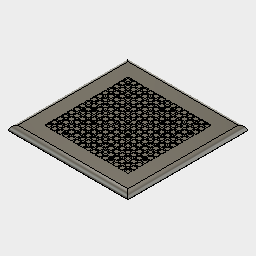
scrabble_board (Autodesk Fusion 360 design; units mm, degrees)
Autodesk Fusion 360 part; units mm, degrees
(part 1 of 6)
sketch "Sketch1" plane through (0, 0, 0) normal (0, 1, 0) x (1, 0, 0)
  line L0 (254, -254) -> (-254, -254)
  line L1 (-254, -254) -> (-254, 254)
  line L2 (-254, 254) -> (254, 254)
  line L3 (254, 254) -> (254, -254)
  line L4 (254, -254) -> (-254, 254) construction
  line L5 (-254, -254) -> (254, 254) construction
  arc A0 (-65.675, -33.5) -> (-62.5, -30.325) centre (-65.675, -30.325) ccw
  line L6 (-65.675, -33.5) -> (-78.325, -33.5)
  dimension "d1" = 508
  dimension "d2" = 508
  constraint perpendicular L0 L1
  constraint parallel L0 L2
  constraint parallel L1 L3
  constraint horizontal L0
  constraint coincident L4 origin
  constraint coincident L5 origin
extrude "Extrude1" add sketch "Sketch1" along normal blind 20.5994
sketch "Sketch2" plane through (0, 20.5994, 0) normal (0, 1, 0) x (-1, 0, 0)
  line L0 (-254, -254) -> (254, -254)
  line L1 (254, -254) -> (254, 254)
  line L2 (254, 254) -> (-254, 254)
  line L3 (-254, 254) -> (-254, -254)
  line L4 (-6.325, 9.5) -> (6.325, 9.5)
  line L5 (9.5, 6.325) -> (9.5, -6.325)
  line L6 (6.325, -9.5) -> (-6.325, -9.5)
  line L7 (-9.5, -6.325) -> (-9.5, 6.325)
  line L8 (-9.5, 9.5) -> (9.5, -9.5) construction
  line L9 (9.5, 9.5) -> (-9.5, -9.5) construction
  arc A0 (6.325, -9.5) -> (9.5, -6.325) centre (6.325, -6.325) ccw
  arc A1 (-9.5, -6.325) -> (-6.325, -9.5) centre (-6.325, -6.325) ccw
  arc A2 (-6.325, 9.5) -> (-9.5, 6.325) centre (-6.325, 6.325) ccw
  arc A3 (9.5, 6.325) -> (6.325, 9.5) centre (6.325, 6.325) ccw
  arc A4 (-161.675, -177.5) -> (-158.5, -174.325) centre (-161.675, -174.325) ccw
  line L10 (-177.5, -174.325) -> (-177.5, -161.675)
  line L11 (-158.5, -161.675) -> (-158.5, -174.325)
  line L12 (-158.5, -158.5) -> (-177.5, -177.5) construction
  arc A5 (-174.325, -158.5) -> (-177.5, -161.675) centre (-174.325, -161.675) ccw
  arc A6 (-158.5, -161.675) -> (-161.675, -158.5) centre (-161.675, -161.675) ccw
  line L13 (-161.675, -177.5) -> (-174.325, -177.5)
  line L14 (-174.325, -158.5) -> (-161.675, -158.5)
  arc A7 (-177.5, -174.325) -> (-174.325, -177.5) centre (-174.325, -174.325) ccw
  line L15 (-177.5, -158.5) -> (-158.5, -177.5) construction
  arc A8 (-137.675, -177.5) -> (-134.5, -174.325) centre (-137.675, -174.325) ccw
  line L16 (-153.5, -174.325) -> (-153.5, -161.675)
  line L17 (-134.5, -161.675) -> (-134.5, -174.325)
  line L18 (-134.5, -158.5) -> (-153.5, -177.5) construction
  arc A9 (-150.325, -158.5) -> (-153.5, -161.675) centre (-150.325, -161.675) ccw
  arc A10 (-134.5, -161.675) -> (-137.675, -158.5) centre (-137.675, -161.675) ccw
  line L19 (-137.675, -177.5) -> (-150.325, -177.5)
  line L20 (-150.325, -158.5) -> (-137.675, -158.5)
  arc A11 (-153.5, -174.325) -> (-150.325, -177.5) centre (-150.325, -174.325) ccw
  line L21 (-153.5, -158.5) -> (-134.5, -177.5) construction
  arc A12 (-113.675, -177.5) -> (-110.5, -174.325) centre (-113.675, -174.325) ccw
  line L22 (-129.5, -174.325) -> (-129.5, -161.675)
  line L23 (-110.5, -161.675) -> (-110.5, -174.325)
  line L24 (-110.5, -158.5) -> (-129.5, -177.5) construction
  arc A13 (-126.325, -158.5) -> (-129.5, -161.675) centre (-126.325, -161.675) ccw
  arc A14 (-110.5, -161.675) -> (-113.675, -158.5) centre (-113.675, -161.675) ccw
  line L25 (-113.675, -177.5) -> (-126.325, -177.5)
  line L26 (-126.325, -158.5) -> (-113.675, -158.5)
  arc A15 (-129.5, -174.325) -> (-126.325, -177.5) centre (-126.325, -174.325) ccw
  line L27 (-129.5, -158.5) -> (-110.5, -177.5) construction
  arc A16 (-89.675, -177.5) -> (-86.5, -174.325) centre (-89.675, -174.325) ccw
  line L28 (-105.5, -174.325) -> (-105.5, -161.675)
  line L29 (-86.5, -161.675) -> (-86.5, -174.325)
  line L30 (-86.5, -158.5) -> (-105.5, -177.5) construction
  arc A17 (-102.325, -158.5) -> (-105.5, -161.675) centre (-102.325, -161.675) ccw
  arc A18 (-86.5, -161.675) -> (-89.675, -158.5) centre (-89.675, -161.675) ccw
  line L31 (-89.675, -177.5) -> (-102.325, -177.5)
  line L32 (-102.325, -158.5) -> (-89.675, -158.5)
  arc A19 (-105.5, -174.325) -> (-102.325, -177.5) centre (-102.325, -174.325) ccw
  line L33 (-105.5, -158.5) -> (-86.5, -177.5) construction
  arc A20 (-65.675, -177.5) -> (-62.5, -174.325) centre (-65.675, -174.325) ccw
  line L34 (-81.5, -174.325) -> (-81.5, -161.675)
  line L35 (-62.5, -161.675) -> (-62.5, -174.325)
  line L36 (-62.5, -158.5) -> (-81.5, -177.5) construction
  arc A21 (-78.325, -158.5) -> (-81.5, -161.675) centre (-78.325, -161.675) ccw
  arc A22 (-62.5, -161.675) -> (-65.675, -158.5) centre (-65.675, -161.675) ccw
  line L37 (-65.675, -177.5) -> (-78.325, -177.5)
  line L38 (-78.325, -158.5) -> (-65.675, -158.5)
  arc A23 (-81.5, -174.325) -> (-78.325, -177.5) centre (-78.325, -174.325) ccw
  line L39 (-81.5, -158.5) -> (-62.5, -177.5) construction
  arc A24 (-41.675, -177.5) -> (-38.5, -174.325) centre (-41.675, -174.325) ccw
  line L40 (-57.5, -174.325) -> (-57.5, -161.675)
  line L41 (-38.5, -161.675) -> (-38.5, -174.325)
  line L42 (-38.5, -158.5) -> (-57.5, -177.5) construction
  arc A25 (-54.325, -158.5) -> (-57.5, -161.675) centre (-54.325, -161.675) ccw
  arc A26 (-38.5, -161.675) -> (-41.675, -158.5) centre (-41.675, -161.675) ccw
  line L43 (-41.675, -177.5) -> (-54.325, -177.5)
  line L44 (-54.325, -158.5) -> (-41.675, -158.5)
  arc A27 (-57.5, -174.325) -> (-54.325, -177.5) centre (-54.325, -174.325) ccw
  line L45 (-57.5, -158.5) -> (-38.5, -177.5) construction
  arc A28 (-17.675, -177.5) -> (-14.5, -174.325) centre (-17.675, -174.325) ccw
  line L46 (-33.5, -174.325) -> (-33.5, -161.675)
  line L47 (-14.5, -161.675) -> (-14.5, -174.325)
  line L48 (-14.5, -158.5) -> (-33.5, -177.5) construction
  arc A29 (-30.325, -158.5) -> (-33.5, -161.675) centre (-30.325, -161.675) ccw
  arc A30 (-14.5, -161.675) -> (-17.675, -158.5) centre (-17.675, -161.675) ccw
  line L49 (-17.675, -177.5) -> (-30.325, -177.5)
  line L50 (-30.325, -158.5) -> (-17.675, -158.5)
  arc A31 (-33.5, -174.325) -> (-30.325, -177.5) centre (-30.325, -174.325) ccw
  line L51 (-33.5, -158.5) -> (-14.5, -177.5) construction
  arc A32 (6.325, -177.5) -> (9.5, -174.325) centre (6.325, -174.325) ccw
  line L52 (-9.5, -174.325) -> (-9.5, -161.675)
  line L53 (9.5, -161.675) -> (9.5, -174.325)
  line L54 (9.5, -158.5) -> (-9.5, -177.5) construction
  arc A33 (-6.325, -158.5) -> (-9.5, -161.675) centre (-6.325, -161.675) ccw
  arc A34 (9.5, -161.675) -> (6.325, -158.5) centre (6.325, -161.675) ccw
  line L55 (6.325, -177.5) -> (-6.325, -177.5)
  line L56 (-6.325, -158.5) -> (6.325, -158.5)
  arc A35 (-9.5, -174.325) -> (-6.325, -177.5) centre (-6.325, -174.325) ccw
  line L57 (-9.5, -158.5) -> (9.5, -177.5) construction
  arc A36 (30.325, -177.5) -> (33.5, -174.325) centre (30.325, -174.325) ccw
  line L58 (14.5, -174.325) -> (14.5, -161.675)
  line L59 (33.5, -161.675) -> (33.5, -174.325)
  line L60 (33.5, -158.5) -> (14.5, -177.5) construction
  arc A37 (17.675, -158.5) -> (14.5, -161.675) centre (17.675, -161.675) ccw
  arc A38 (33.5, -161.675) -> (30.325, -158.5) centre (30.325, -161.675) ccw
  line L61 (30.325, -177.5) -> (17.675, -177.5)
  line L62 (17.675, -158.5) -> (30.325, -158.5)
  arc A39 (14.5, -174.325) -> (17.675, -177.5) centre (17.675, -174.325) ccw
  line L63 (14.5, -158.5) -> (33.5, -177.5) construction
  arc A40 (54.325, -177.5) -> (57.5, -174.325) centre (54.325, -174.325) ccw
  line L64 (38.5, -174.325) -> (38.5, -161.675)
  line L65 (57.5, -161.675) -> (57.5, -174.325)
  line L66 (57.5, -158.5) -> (38.5, -177.5) construction
  arc A41 (41.675, -158.5) -> (38.5, -161.675) centre (41.675, -161.675) ccw
  arc A42 (57.5, -161.675) -> (54.325, -158.5) centre (54.325, -161.675) ccw
  line L67 (54.325, -177.5) -> (41.675, -177.5)
  line L68 (41.675, -158.5) -> (54.325, -158.5)
  arc A43 (38.5, -174.325) -> (41.675, -177.5) centre (41.675, -174.325) ccw
  line L69 (38.5, -158.5) -> (57.5, -177.5) construction
  arc A44 (78.325, -177.5) -> (81.5, -174.325) centre (78.325, -174.325) ccw
  line L70 (62.5, -174.325) -> (62.5, -161.675)
  line L71 (81.5, -161.675) -> (81.5, -174.325)
  line L72 (81.5, -158.5) -> (62.5, -177.5) construction
  arc A45 (65.675, -158.5) -> (62.5, -161.675) centre (65.675, -161.675) ccw
  arc A46 (81.5, -161.675) -> (78.325, -158.5) centre (78.325, -161.675) ccw
  line L73 (78.325, -177.5) -> (65.675, -177.5)
  line L74 (65.675, -158.5) -> (78.325, -158.5)
  arc A47 (62.5, -174.325) -> (65.675, -177.5) centre (65.675, -174.325) ccw
  line L75 (62.5, -158.5) -> (81.5, -177.5) construction
  arc A48 (102.325, -177.5) -> (105.5, -174.325) centre (102.325, -174.325) ccw
  line L76 (86.5, -174.325) -> (86.5, -161.675)
  line L77 (105.5, -161.675) -> (105.5, -174.325)
  line L78 (105.5, -158.5) -> (86.5, -177.5) construction
  arc A49 (89.675, -158.5) -> (86.5, -161.675) centre (89.675, -161.675) ccw
  arc A50 (105.5, -161.675) -> (102.325, -158.5) centre (102.325, -161.675) ccw
  line L79 (102.325, -177.5) -> (89.675, -177.5)
  line L80 (89.675, -158.5) -> (102.325, -158.5)
  arc A51 (86.5, -174.325) -> (89.675, -177.5) centre (89.675, -174.325) ccw
  line L81 (86.5, -158.5) -> (105.5, -177.5) construction
  arc A52 (126.325, -177.5) -> (129.5, -174.325) centre (126.325, -174.325) ccw
  line L82 (110.5, -174.325) -> (110.5, -161.675)
  line L83 (129.5, -161.675) -> (129.5, -174.325)
  line L84 (129.5, -158.5) -> (110.5, -177.5) construction
  arc A53 (113.675, -158.5) -> (110.5, -161.675) centre (113.675, -161.675) ccw
  arc A54 (129.5, -161.675) -> (126.325, -158.5) centre (126.325, -161.675) ccw
  line L85 (126.325, -177.5) -> (113.675, -177.5)
  line L86 (113.675, -158.5) -> (126.325, -158.5)
  arc A55 (110.5, -174.325) -> (113.675, -177.5) centre (113.675, -174.325) ccw
  line L87 (110.5, -158.5) -> (129.5, -177.5) construction
  arc A56 (150.325, -177.5) -> (153.5, -174.325) centre (150.325, -174.325) ccw
  line L88 (134.5, -174.325) -> (134.5, -161.675)
  line L89 (153.5, -161.675) -> (153.5, -174.325)
  line L90 (153.5, -158.5) -> (134.5, -177.5) construction
  arc A57 (137.675, -158.5) -> (134.5, -161.675) centre (137.675, -161.675) ccw
  arc A58 (153.5, -161.675) -> (150.325, -158.5) centre (150.325, -161.675) ccw
  line L91 (150.325, -177.5) -> (137.675, -177.5)
  line L92 (137.675, -158.5) -> (150.325, -158.5)
  arc A59 (134.5, -174.325) -> (137.675, -177.5) centre (137.675, -174.325) ccw
  line L93 (134.5, -158.5) -> (153.5, -177.5) construction
  arc A60 (174.325, -177.5) -> (177.5, -174.325) centre (174.325, -174.325) ccw
  line L94 (158.5, -174.325) -> (158.5, -161.675)
  line L95 (177.5, -161.675) -> (177.5, -174.325)
  line L96 (177.5, -158.5) -> (158.5, -177.5) construction
  arc A61 (161.675, -158.5) -> (158.5, -161.675) centre (161.675, -161.675) ccw
  arc A62 (177.5, -161.675) -> (174.325, -158.5) centre (174.325, -161.675) ccw
  line L97 (174.325, -177.5) -> (161.675, -177.5)
  line L98 (161.675, -158.5) -> (174.325, -158.5)
  arc A63 (158.5, -174.325) -> (161.675, -177.5) centre (161.675, -174.325) ccw
  line L99 (158.5, -158.5) -> (177.5, -177.5) construction
  arc A64 (-161.675, -153.5) -> (-158.5, -150.325) centre (-161.675, -150.325) ccw
  line L100 (-177.5, -150.325) -> (-177.5, -137.675)
  line L101 (-158.5, -137.675) -> (-158.5, -150.325)
  line L102 (-158.5, -134.5) -> (-177.5, -153.5) construction
  arc A65 (-174.325, -134.5) -> (-177.5, -137.675) centre (-174.325, -137.675) ccw
  arc A66 (-158.5, -137.675) -> (-161.675, -134.5) centre (-161.675, -137.675) ccw
  line L103 (-161.675, -153.5) -> (-174.325, -153.5)
  line L104 (-174.325, -134.5) -> (-161.675, -134.5)
  arc A67 (-177.5, -150.325) -> (-174.325, -153.5) centre (-174.325, -150.325) ccw
  line L105 (-177.5, -134.5) -> (-158.5, -153.5) construction
  arc A68 (-137.675, -153.5) -> (-134.5, -150.325) centre (-137.675, -150.325) ccw
  line L106 (-153.5, -150.325) -> (-153.5, -137.675)
  line L107 (-134.5, -137.675) -> (-134.5, -150.325)
  line L108 (-134.5, -134.5) -> (-153.5, -153.5) construction
  arc A69 (-150.325, -134.5) -> (-153.5, -137.675) centre (-150.325, -137.675) ccw
  arc A70 (-134.5, -137.675) -> (-137.675, -134.5) centre (-137.675, -137.675) ccw
  line L109 (-137.675, -153.5) -> (-150.325, -153.5)
  line L110 (-150.325, -134.5) -> (-137.675, -134.5)
  arc A71 (-153.5, -150.325) -> (-150.325, -153.5) centre (-150.325, -150.325) ccw
  line L111 (-153.5, -134.5) -> (-134.5, -153.5) construction
  arc A72 (-113.675, -153.5) -> (-110.5, -150.325) centre (-113.675, -150.325) ccw
  line L112 (-129.5, -150.325) -> (-129.5, -137.675)
  line L113 (-110.5, -137.675) -> (-110.5, -150.325)
  line L114 (-110.5, -134.5) -> (-129.5, -153.5) construction
  arc A73 (-126.325, -134.5) -> (-129.5, -137.675) centre (-126.325, -137.675) ccw
  arc A74 (-110.5, -137.675) -> (-113.675, -134.5) centre (-113.675, -137.675) ccw
  line L115 (-113.675, -153.5) -> (-126.325, -153.5)
  line L116 (-126.325, -134.5) -> (-113.675, -134.5)
  arc A75 (-129.5, -150.325) -> (-126.325, -153.5) centre (-126.325, -150.325) ccw
  line L117 (-129.5, -134.5) -> (-110.5, -153.5) construction
  arc A76 (-89.675, -153.5) -> (-86.5, -150.325) centre (-89.675, -150.325) ccw
  line L118 (-105.5, -150.325) -> (-105.5, -137.675)
  line L119 (-86.5, -137.675) -> (-86.5, -150.325)
  line L120 (-86.5, -134.5) -> (-105.5, -153.5) construction
  arc A77 (-102.325, -134.5) -> (-105.5, -137.675) centre (-102.325, -137.675) ccw
  arc A78 (-86.5, -137.675) -> (-89.675, -134.5) centre (-89.675, -137.675) ccw
  line L121 (-89.675, -153.5) -> (-102.325, -153.5)
  line L122 (-102.325, -134.5) -> (-89.675, -134.5)
  arc A79 (-105.5, -150.325) -> (-102.325, -153.5) centre (-102.325, -150.325) ccw
  line L123 (-105.5, -134.5) -> (-86.5, -153.5) construction
  arc A80 (-65.675, -153.5) -> (-62.5, -150.325) centre (-65.675, -150.325) ccw
  line L124 (-81.5, -150.325) -> (-81.5, -137.675)
  line L125 (-62.5, -137.675) -> (-62.5, -150.325)
  line L126 (-62.5, -134.5) -> (-81.5, -153.5) construction
  arc A81 (-78.325, -134.5) -> (-81.5, -137.675) centre (-78.325, -137.675) ccw
  arc A82 (-62.5, -137.675) -> (-65.675, -134.5) centre (-65.675, -137.675) ccw
  line L127 (-65.675, -153.5) -> (-78.325, -153.5)
  line L128 (-78.325, -134.5) -> (-65.675, -134.5)
  arc A83 (-81.5, -150.325) -> (-78.325, -153.5) centre (-78.325, -150.325) ccw
  line L129 (-81.5, -134.5) -> (-62.5, -153.5) construction
  arc A84 (-41.675, -153.5) -> (-38.5, -150.325) centre (-41.675, -150.325) ccw
  line L130 (-57.5, -150.325) -> (-57.5, -137.675)
  line L131 (-38.5, -137.675) -> (-38.5, -150.325)
  line L132 (-38.5, -134.5) -> (-57.5, -153.5) construction
  arc A85 (-54.325, -134.5) -> (-57.5, -137.675) centre (-54.325, -137.675) ccw
  arc A86 (-38.5, -137.675) -> (-41.675, -134.5) centre (-41.675, -137.675) ccw
  line L133 (-41.675, -153.5) -> (-54.325, -153.5)
  line L134 (-54.325, -134.5) -> (-41.675, -134.5)
  arc A87 (-57.5, -150.325) -> (-54.325, -153.5) centre (-54.325, -150.325) ccw
  line L135 (-57.5, -134.5) -> (-38.5, -153.5) construction
  arc A88 (-17.675, -153.5) -> (-14.5, -150.325) centre (-17.675, -150.325) ccw
  line L136 (-33.5, -150.325) -> (-33.5, -137.675)
  line L137 (-14.5, -137.675) -> (-14.5, -150.325)
  line L138 (-14.5, -134.5) -> (-33.5, -153.5) construction
  arc A89 (-30.325, -134.5) -> (-33.5, -137.675) centre (-30.325, -137.675) ccw
  arc A90 (-14.5, -137.675) -> (-17.675, -134.5) centre (-17.675, -137.675) ccw
  line L139 (-17.675, -153.5) -> (-30.325, -153.5)
  line L140 (-30.325, -134.5) -> (-17.675, -134.5)
  arc A91 (-33.5, -150.325) -> (-30.325, -153.5) centre (-30.325, -150.325) ccw
  line L141 (-33.5, -134.5) -> (-14.5, -153.5) construction
  arc A92 (6.325, -153.5) -> (9.5, -150.325) centre (6.325, -150.325) ccw
  line L142 (-9.5, -150.325) -> (-9.5, -137.675)
  line L143 (9.5, -137.675) -> (9.5, -150.325)
  line L144 (9.5, -134.5) -> (-9.5, -153.5) construction
  arc A93 (-6.325, -134.5) -> (-9.5, -137.675) centre (-6.325, -137.675) ccw
  arc A94 (9.5, -137.675) -> (6.325, -134.5) centre (6.325, -137.675) ccw
  line L145 (6.325, -153.5) -> (-6.325, -153.5)
  line L146 (-6.325, -134.5) -> (6.325, -134.5)
  arc A95 (-9.5, -150.325) -> (-6.325, -153.5) centre (-6.325, -150.325) ccw
  line L147 (-9.5, -134.5) -> (9.5, -153.5) construction
  arc A96 (30.325, -153.5) -> (33.5, -150.325) centre (30.325, -150.325) ccw
  line L148 (14.5, -150.325) -> (14.5, -137.675)
  line L149 (33.5, -137.675) -> (33.5, -150.325)
  line L150 (33.5, -134.5) -> (14.5, -153.5) construction
  arc A97 (17.675, -134.5) -> (14.5, -137.675) centre (17.675, -137.675) ccw
  arc A98 (33.5, -137.675) -> (30.325, -134.5) centre (30.325, -137.675) ccw
  line L151 (30.325, -153.5) -> (17.675, -153.5)
  line L152 (17.675, -134.5) -> (30.325, -134.5)
  arc A99 (14.5, -150.325) -> (17.675, -153.5) centre (17.675, -150.325) ccw
  line L153 (14.5, -134.5) -> (33.5, -153.5) construction
  arc A100 (54.325, -153.5) -> (57.5, -150.325) centre (54.325, -150.325) ccw
  line L154 (38.5, -150.325) -> (38.5, -137.675)
  line L155 (57.5, -137.675) -> (57.5, -150.325)
  line L156 (57.5, -134.5) -> (38.5, -153.5) construction
  arc A101 (41.675, -134.5) -> (38.5, -137.675) centre (41.675, -137.675) ccw
  arc A102 (57.5, -137.675) -> (54.325, -134.5) centre (54.325, -137.675) ccw
  line L157 (54.325, -153.5) -> (41.675, -153.5)
  line L158 (41.675, -134.5) -> (54.325, -134.5)
  arc A103 (38.5, -150.325) -> (41.675, -153.5) centre (41.675, -150.325) ccw
  line L159 (38.5, -134.5) -> (57.5, -153.5) construction
  arc A104 (78.325, -153.5) -> (81.5, -150.325) centre (78.325, -150.325) ccw
  line L160 (62.5, -150.325) -> (62.5, -137.675)
  line L161 (81.5, -137.675) -> (81.5, -150.325)
  line L162 (81.5, -134.5) -> (62.5, -153.5) construction
  arc A105 (65.675, -134.5) -> (62.5, -137.675) centre (65.675, -137.675) ccw
  arc A106 (81.5, -137.675) -> (78.325, -134.5) centre (78.325, -137.675) ccw
  line L163 (78.325, -153.5) -> (65.675, -153.5)
  line L164 (65.675, -134.5) -> (78.325, -134.5)
  arc A107 (62.5, -150.325) -> (65.675, -153.5) centre (65.675, -150.325) ccw
  line L165 (62.5, -134.5) -> (81.5, -153.5) construction
  arc A108 (102.325, -153.5) -> (105.5, -150.325) centre (102.325, -150.325) ccw
  line L166 (86.5, -150.325) -> (86.5, -137.675)
  line L167 (105.5, -137.675) -> (105.5, -150.325)
  line L168 (105.5, -134.5) -> (86.5, -153.5) construction
  arc A109 (89.675, -134.5) -> (86.5, -137.675) centre (89.675, -137.675) ccw
  arc A110 (105.5, -137.675) -> (102.325, -134.5) centre (102.325, -137.675) ccw
  line L169 (102.325, -153.5) -> (89.675, -153.5)
  line L170 (89.675, -134.5) -> (102.325, -134.5)
  arc A111 (86.5, -150.325) -> (89.675, -153.5) centre (89.675, -150.325) ccw
  line L171 (86.5, -134.5) -> (105.5, -153.5) construction
  arc A112 (126.325, -153.5) -> (129.5, -150.325) centre (126.325, -150.325) ccw
  line L172 (110.5, -150.325) -> (110.5, -137.675)
  line L173 (129.5, -137.675) -> (129.5, -150.325)
  line L174 (129.5, -134.5) -> (110.5, -153.5) construction
  arc A113 (113.675, -134.5) -> (110.5, -137.675) centre (113.675, -137.675) ccw
  arc A114 (129.5, -137.675) -> (126.325, -134.5) centre (126.325, -137.675) ccw
  line L175 (126.325, -153.5) -> (113.675, -153.5)
  line L176 (113.675, -134.5) -> (126.325, -134.5)
  arc A115 (110.5, -150.325) -> (113.675, -153.5) centre (113.675, -150.325) ccw
  line L177 (110.5, -134.5) -> (129.5, -153.5) construction
  arc A116 (150.325, -153.5) -> (153.5, -150.325) centre (150.325, -150.325) ccw
  line L178 (134.5, -150.325) -> (134.5, -137.675)
  line L179 (153.5, -137.675) -> (153.5, -150.325)
  line L180 (153.5, -134.5) -> (134.5, -153.5) construction
  arc A117 (137.675, -134.5) -> (134.5, -137.675) centre (137.675, -137.675) ccw
  arc A118 (153.5, -137.675) -> (150.325, -134.5) centre (150.325, -137.675) ccw
  line L181 (150.325, -153.5) -> (137.675, -153.5)
  line L182 (137.675, -134.5) -> (150.325, -134.5)
  arc A119 (134.5, -150.325) -> (137.675, -153.5) centre (137.675, -150.325) ccw
  line L183 (134.5, -134.5) -> (153.5, -153.5) construction
  arc A120 (174.325, -153.5) -> (177.5, -150.325) centre (174.325, -150.325) ccw
  line L184 (158.5, -150.325) -> (158.5, -137.675)
  line L185 (177.5, -137.675) -> (177.5, -150.325)
  line L186 (177.5, -134.5) -> (158.5, -153.5) construction
  arc A121 (161.675, -134.5) -> (158.5, -137.675) centre (161.675, -137.675) ccw
  arc A122 (177.5, -137.675) -> (174.325, -134.5) centre (174.325, -137.675) ccw
  line L187 (174.325, -153.5) -> (161.675, -153.5)
  line L188 (161.675, -134.5) -> (174.325, -134.5)
  arc A123 (158.5, -150.325) -> (161.675, -153.5) centre (161.675, -150.325) ccw
  line L189 (158.5, -134.5) -> (177.5, -153.5) construction
  arc A124 (-161.675, -129.5) -> (-158.5, -126.325) centre (-161.675, -126.325) ccw
  line L190 (-177.5, -126.325) -> (-177.5, -113.675)
  line L191 (-158.5, -113.675) -> (-158.5, -126.325)
  line L192 (-158.5, -110.5) -> (-177.5, -129.5) construction
  arc A125 (-174.325, -110.5) -> (-177.5, -113.675) centre (-174.325, -113.675) ccw
  arc A126 (-158.5, -113.675) -> (-161.675, -110.5) centre (-161.675, -113.675) ccw
  line L193 (-161.675, -129.5) -> (-174.325, -129.5)
  line L194 (-174.325, -110.5) -> (-161.675, -110.5)
  arc A127 (-177.5, -126.325) -> (-174.325, -129.5) centre (-174.325, -126.325) ccw
  line L195 (-177.5, -110.5) -> (-158.5, -129.5) construction
  arc A128 (-137.675, -129.5) -> (-134.5, -126.325) centre (-137.675, -126.325) ccw
  line L196 (-153.5, -126.325) -> (-153.5, -113.675)
  line L197 (-134.5, -113.675) -> (-134.5, -126.325)
  line L198 (-134.5, -110.5) -> (-153.5, -129.5) construction
  arc A129 (-150.325, -110.5) -> (-153.5, -113.675) centre (-150.325, -113.675) ccw
  arc A130 (-134.5, -113.675) -> (-137.675, -110.5) centre (-137.675, -113.675) ccw
  line L199 (-137.675, -129.5) -> (-150.325, -129.5)
  line L200 (-150.325, -110.5) -> (-137.675, -110.5)
  arc A131 (-153.5, -126.325) -> (-150.325, -129.5) centre (-150.325, -126.325) ccw
  line L201 (-153.5, -110.5) -> (-134.5, -129.5) construction
  arc A132 (-113.675, -129.5) -> (-110.5, -126.325) centre (-113.675, -126.325) ccw
  line L202 (-129.5, -126.325) -> (-129.5, -113.675)
  line L203 (-110.5, -113.675) -> (-110.5, -126.325)
  line L204 (-110.5, -110.5) -> (-129.5, -129.5) construction
  arc A133 (-126.325, -110.5) -> (-129.5, -113.675) centre (-126.325, -113.675) ccw
  arc A134 (-110.5, -113.675) -> (-113.675, -110.5) centre (-113.675, -113.675) ccw
  line L205 (-113.675, -129.5) -> (-126.325, -129.5)
  line L206 (-126.325, -110.5) -> (-113.675, -110.5)
  arc A135 (-129.5, -126.325) -> (-126.325, -129.5) centre (-126.325, -126.325) ccw
  line L207 (-129.5, -110.5) -> (-110.5, -129.5) construction
  arc A136 (-89.675, -129.5) -> (-86.5, -126.325) centre (-89.675, -126.325) ccw
  line L208 (-105.5, -126.325) -> (-105.5, -113.675)
  line L209 (-86.5, -113.675) -> (-86.5, -126.325)
  line L210 (-86.5, -110.5) -> (-105.5, -129.5) construction
  arc A137 (-102.325, -110.5) -> (-105.5, -113.675) centre (-102.325, -113.675) ccw
  arc A138 (-86.5, -113.675) -> (-89.675, -110.5) centre (-89.675, -113.675) ccw
  line L211 (-89.675, -129.5) -> (-102.325, -129.5)
  line L212 (-102.325, -110.5) -> (-89.675, -110.5)
  arc A139 (-105.5, -126.325) -> (-102.325, -129.5) centre (-102.325, -126.325) ccw
  line L213 (-105.5, -110.5) -> (-86.5, -129.5) construction
  arc A140 (-65.675, -129.5) -> (-62.5, -126.325) centre (-65.675, -126.325) ccw
  line L214 (-81.5, -126.325) -> (-81.5, -113.675)
  line L215 (-62.5, -113.675) -> (-62.5, -126.325)
  line L216 (-62.5, -110.5) -> (-81.5, -129.5) construction
  arc A141 (-78.325, -110.5) -> (-81.5, -113.675) centre (-78.325, -113.675) ccw
  arc A142 (-62.5, -113.675) -> (-65.675, -110.5) centre (-65.675, -113.675) ccw
  line L217 (-65.675, -129.5) -> (-78.325, -129.5)
  line L218 (-78.325, -110.5) -> (-65.675, -110.5)
  arc A143 (-81.5, -126.325) -> (-78.325, -129.5) centre (-78.325, -126.325) ccw
  line L219 (-81.5, -110.5) -> (-62.5, -129.5) construction
  arc A144 (-41.675, -129.5) -> (-38.5, -126.325) centre (-41.675, -126.325) ccw
  line L220 (-57.5, -126.325) -> (-57.5, -113.675)
  line L221 (-38.5, -113.675) -> (-38.5, -126.325)
  line L222 (-38.5, -110.5) -> (-57.5, -129.5) construction
  arc A145 (-54.325, -110.5) -> (-57.5, -113.675) centre (-54.325, -113.675) ccw
  arc A146 (-38.5, -113.675) -> (-41.675, -110.5) centre (-41.675, -113.675) ccw
  line L223 (-41.675, -129.5) -> (-54.325, -129.5)
  line L224 (-54.325, -110.5) -> (-41.675, -110.5)
  arc A147 (-57.5, -126.325) -> (-54.325, -129.5) centre (-54.325, -126.325) ccw
  line L225 (-57.5, -110.5) -> (-38.5, -129.5) construction
  arc A148 (-17.675, -129.5) -> (-14.5, -126.325) centre (-17.675, -126.325) ccw
  line L226 (-33.5, -126.325) -> (-33.5, -113.675)
  line L227 (-14.5, -113.675) -> (-14.5, -126.325)
  line L228 (-14.5, -110.5) -> (-33.5, -129.5) construction
  arc A149 (-30.325, -110.5) -> (-33.5, -113.675) centre (-30.325, -113.675) ccw
  arc A150 (-14.5, -113.675) -> (-17.675, -110.5) centre (-17.675, -113.675) ccw
  line L229 (-17.675, -129.5) -> (-30.325, -129.5)
  line L230 (-30.325, -110.5) -> (-17.675, -110.5)
  arc A151 (-33.5, -126.325) -> (-30.325, -129.5) centre (-30.325, -126.325) ccw
  line L231 (-33.5, -110.5) -> (-14.5, -129.5) construction
  arc A152 (6.325, -129.5) -> (9.5, -126.325) centre (6.325, -126.325) ccw
  line L232 (-9.5, -126.325) -> (-9.5, -113.675)
  line L233 (9.5, -113.675) -> (9.5, -126.325)
  line L234 (9.5, -110.5) -> (-9.5, -129.5) construction
  arc A153 (-6.325, -110.5) -> (-9.5, -113.675) centre (-6.325, -113.675) ccw
  arc A154 (9.5, -113.675) -> (6.325, -110.5) centre (6.325, -113.675) ccw
  line L235 (6.325, -129.5) -> (-6.325, -129.5)
  line L236 (-6.325, -110.5) -> (6.325, -110.5)
  arc A155 (-9.5, -126.325) -> (-6.325, -129.5) centre (-6.325, -126.325) ccw
  line L237 (-9.5, -110.5) -> (9.5, -129.5) construction
  arc A156 (30.325, -129.5) -> (33.5, -126.325) centre (30.325, -126.325) ccw
  line L238 (14.5, -126.325) -> (14.5, -113.675)
  line L239 (33.5, -113.675) -> (33.5, -126.325)
  line L240 (33.5, -110.5) -> (14.5, -129.5) construction
  arc A157 (17.675, -110.5) -> (14.5, -113.675) centre (17.675, -113.675) ccw
  arc A158 (33.5, -113.675) -> (30.325, -110.5) centre (30.325, -113.675) ccw
  line L241 (30.325, -129.5) -> (17.675, -129.5)
  line L242 (17.675, -110.5) -> (30.325, -110.5)
  arc A159 (14.5, -126.325) -> (17.675, -129.5) centre (17.675, -126.325) ccw
  line L243 (14.5, -110.5) -> (33.5, -129.5) construction
  arc A160 (54.325, -129.5) -> (57.5, -126.325) centre (54.325, -126.325) ccw
  line L244 (38.5, -126.325) -> (38.5, -113.675)
  line L245 (57.5, -113.675) -> (57.5, -126.325)
  line L246 (57.5, -110.5) -> (38.5, -129.5) construction
  arc A161 (41.675, -110.5) -> (38.5, -113.675) centre (41.675, -113.675) ccw
  arc A162 (57.5, -113.675) -> (54.325, -110.5) centre (54.325, -113.675) ccw
  line L247 (54.325, -129.5) -> (41.675, -129.5)
  line L248 (41.675, -110.5) -> (54.325, -110.5)
  arc A163 (38.5, -126.325) -> (41.675, -129.5) centre (41.675, -126.325) ccw
  line L249 (38.5, -110.5) -> (57.5, -129.5) construction
  arc A164 (78.325, -129.5) -> (81.5, -126.325) centre (78.325, -126.325) ccw
  line L250 (62.5, -126.325) -> (62.5, -113.675)
  line L251 (81.5, -113.675) -> (81.5, -126.325)
  line L252 (81.5, -110.5) -> (62.5, -129.5) construction
  arc A165 (65.675, -110.5) -> (62.5, -113.675) centre (65.675, -113.675) ccw
  arc A166 (81.5, -113.675) -> (78.325, -110.5) centre (78.325, -113.675) ccw
  line L253 (78.325, -129.5) -> (65.675, -129.5)
  line L254 (65.675, -110.5) -> (78.325, -110.5)
  arc A167 (62.5, -126.325) -> (65.675, -129.5) centre (65.675, -126.325) ccw
  line L255 (62.5, -110.5) -> (81.5, -129.5) construction
  arc A168 (102.325, -129.5) -> (105.5, -126.325) centre (102.325, -126.325) ccw
  line L256 (86.5, -126.325) -> (86.5, -113.675)
  line L257 (105.5, -113.675) -> (105.5, -126.325)
  line L258 (105.5, -110.5) -> (86.5, -129.5) construction
  arc A169 (89.675, -110.5) -> (86.5, -113.675) centre (89.675, -113.675) ccw
  arc A170 (105.5, -113.675) -> (102.325, -110.5) centre (102.325, -113.675) ccw
  line L259 (102.325, -129.5) -> (89.675, -129.5)
  line L260 (89.675, -110.5) -> (102.325, -110.5)
  arc A171 (86.5, -126.325) -> (89.675, -129.5) centre (89.675, -126.325) ccw
  line L261 (86.5, -110.5) -> (105.5, -129.5) construction
  arc A172 (126.325, -129.5) -> (129.5, -126.325) centre (126.325, -126.325) ccw
  line L262 (110.5, -126.325) -> (110.5, -113.675)
  line L263 (129.5, -113.675) -> (129.5, -126.325)
  line L264 (129.5, -110.5) -> (110.5, -129.5) construction
  arc A173 (113.675, -110.5) -> (110.5, -113.675) centre (113.675, -113.675) ccw
  arc A174 (129.5, -113.675) -> (126.325, -110.5) centre (126.325, -113.675) ccw
  line L265 (126.325, -129.5) -> (113.675, -129.5)
  line L266 (113.675, -110.5) -> (126.325, -110.5)
  arc A175 (110.5, -126.325) -> (113.675, -129.5) centre (113.675, -126.325) ccw
  line L267 (110.5, -110.5) -> (129.5, -129.5) construction
  arc A176 (150.325, -129.5) -> (153.5, -126.325) centre (150.325, -126.325) ccw
  line L268 (134.5, -126.325) -> (134.5, -113.675)
  line L269 (153.5, -113.675) -> (153.5, -126.325)
  line L270 (153.5, -110.5) -> (134.5, -129.5) construction
  arc A177 (137.675, -110.5) -> (134.5, -113.675) centre (137.675, -113.675) ccw
  arc A178 (153.5, -113.675) -> (150.325, -110.5) centre (150.325, -113.675) ccw
  line L271 (150.325, -129.5) -> (137.675, -129.5)
  line L272 (137.675, -110.5) -> (150.325, -110.5)
  arc A179 (134.5, -126.325) -> (137.675, -129.5) centre (137.675, -126.325) ccw
  line L273 (134.5, -110.5) -> (153.5, -129.5) construction
  arc A180 (174.325, -129.5) -> (177.5, -126.325) centre (174.325, -126.325) ccw
  line L274 (158.5, -126.325) -> (158.5, -113.675)
  line L275 (177.5, -113.675) -> (177.5, -126.325)
  line L276 (177.5, -110.5) -> (158.5, -129.5) construction
  arc A181 (161.675, -110.5) -> (158.5, -113.675) centre (161.675, -113.675) ccw
  arc A182 (177.5, -113.675) -> (174.325, -110.5) centre (174.325, -113.675) ccw
  line L277 (174.325, -129.5) -> (161.675, -129.5)
  line L278 (161.675, -110.5) -> (174.325, -110.5)
  arc A183 (158.5, -126.325) -> (161.675, -129.5) centre (161.675, -126.325) ccw
  line L279 (158.5, -110.5) -> (177.5, -129.5) construction
  arc A184 (-161.675, -105.5) -> (-158.5, -102.325) centre (-161.675, -102.325) ccw
  line L280 (-177.5, -102.325) -> (-177.5, -89.675)
  line L281 (-158.5, -89.675) -> (-158.5, -102.325)
  line L282 (-158.5, -86.5) -> (-177.5, -105.5) construction
  arc A185 (-174.325, -86.5) -> (-177.5, -89.675) centre (-174.325, -89.675) ccw
  arc A186 (-158.5, -89.675) -> (-161.675, -86.5) centre (-161.675, -89.675) ccw
  line L283 (-161.675, -105.5) -> (-174.325, -105.5)
  line L284 (-174.325, -86.5) -> (-161.675, -86.5)
  arc A187 (-177.5, -102.325) -> (-174.325, -105.5) centre (-174.325, -102.325) ccw
  line L285 (-177.5, -86.5) -> (-158.5, -105.5) construction
  arc A188 (-137.675, -105.5) -> (-134.5, -102.325) centre (-137.675, -102.325) ccw
  line L286 (-153.5, -102.325) -> (-153.5, -89.675)
  line L287 (-134.5, -89.675) -> (-134.5, -102.325)
  line L288 (-134.5, -86.5) -> (-153.5, -105.5) construction
  arc A189 (-150.325, -86.5) -> (-153.5, -89.675) centre (-150.325, -89.675) ccw
  arc A190 (-134.5, -89.675) -> (-137.675, -86.5) centre (-137.675, -89.675) ccw
  line L289 (-137.675, -105.5) -> (-150.325, -105.5)
  line L290 (-150.325, -86.5) -> (-137.675, -86.5)
  arc A191 (-153.5, -102.325) -> (-150.325, -105.5) centre (-150.325, -102.325) ccw
  line L291 (-153.5, -86.5) -> (-134.5, -105.5) construction
  arc A192 (-113.675, -105.5) -> (-110.5, -102.325) centre (-113.675, -102.325) ccw
  line L292 (-129.5, -102.325) -> (-129.5, -89.675)
  line L293 (-110.5, -89.675) -> (-110.5, -102.325)
  line L294 (-110.5, -86.5) -> (-129.5, -105.5) construction
  arc A193 (-126.325, -86.5) -> (-129.5, -89.675) centre (-126.325, -89.675) ccw
  arc A194 (-110.5, -89.675) -> (-113.675, -86.5) centre (-113.675, -89.675) ccw
  line L295 (-113.675, -105.5) -> (-126.325, -105.5)
  line L296 (-126.325, -86.5) -> (-113.675, -86.5)
  arc A195 (-129.5, -102.325) -> (-126.325, -105.5) centre (-126.325, -102.325) ccw
  line L297 (-129.5, -86.5) -> (-110.5, -105.5) construction
  arc A196 (-89.675, -105.5) -> (-86.5, -102.325) centre (-89.675, -102.325) ccw
  line L298 (-105.5, -102.325) -> (-105.5, -89.675)
  line L299 (-86.5, -89.675) -> (-86.5, -102.325)
  line L300 (-86.5, -86.5) -> (-105.5, -105.5) construction
  arc A197 (-102.325, -86.5) -> (-105.5, -89.675) centre (-102.325, -89.675) ccw
  arc A198 (-86.5, -89.675) -> (-89.675, -86.5) centre (-89.675, -89.675) ccw
  line L301 (-89.675, -105.5) -> (-102.325, -105.5)
  line L302 (-102.325, -86.5) -> (-89.675, -86.5)
  arc A199 (-105.5, -102.325) -> (-102.325, -105.5) centre (-102.325, -102.325) ccw
  line L303 (-105.5, -86.5) -> (-86.5, -105.5) construction
  arc A200 (-65.675, -105.5) -> (-62.5, -102.325) centre (-65.675, -102.325) ccw
  line L304 (-81.5, -102.325) -> (-81.5, -89.675)
  line L305 (-62.5, -89.675) -> (-62.5, -102.325)
  line L306 (-62.5, -86.5) -> (-81.5, -105.5) construction
  arc A201 (-78.325, -86.5) -> (-81.5, -89.675) centre (-78.325, -89.675) ccw
  arc A202 (-62.5, -89.675) -> (-65.675, -86.5) centre (-65.675, -89.675) ccw
  line L307 (-65.675, -105.5) -> (-78.325, -105.5)
  line L308 (-78.325, -86.5) -> (-65.675, -86.5)
  arc A203 (-81.5, -102.325) -> (-78.325, -105.5) centre (-78.325, -102.325) ccw
  line L309 (-81.5, -86.5) -> (-62.5, -105.5) construction
  arc A204 (-41.675, -105.5) -> (-38.5, -102.325) centre (-41.675, -102.325) ccw
  line L310 (-57.5, -102.325) -> (-57.5, -89.675)
  line L311 (-38.5, -89.675) -> (-38.5, -102.325)
  line L312 (-38.5, -86.5) -> (-57.5, -105.5) construction
  arc A205 (-54.325, -86.5) -> (-57.5, -89.675) centre (-54.325, -89.675) ccw
  arc A206 (-38.5, -89.675) -> (-41.675, -86.5) centre (-41.675, -89.675) ccw
  line L313 (-41.675, -105.5) -> (-54.325, -105.5)
  line L314 (-54.325, -86.5) -> (-41.675, -86.5)
  arc A207 (-57.5, -102.325) -> (-54.325, -105.5) centre (-54.325, -102.325) ccw
  line L315 (-57.5, -86.5) -> (-38.5, -105.5) construction
  arc A208 (-17.675, -105.5) -> (-14.5, -102.325) centre (-17.675, -102.325) ccw
  line L316 (-33.5, -102.325) -> (-33.5, -89.675)
  line L317 (-14.5, -89.675) -> (-14.5, -102.325)
  line L318 (-14.5, -86.5) -> (-33.5, -105.5) construction
  arc A209 (-30.325, -86.5) -> (-33.5, -89.675) centre (-30.325, -89.675) ccw
  arc A210 (-14.5, -89.675) -> (-17.675, -86.5) centre (-17.675, -89.675) ccw
  line L319 (-17.675, -105.5) -> (-30.325, -105.5)
  line L320 (-30.325, -86.5) -> (-17.675, -86.5)
  arc A211 (-33.5, -102.325) -> (-30.325, -105.5) centre (-30.325, -102.325) ccw
  line L321 (-33.5, -86.5) -> (-14.5, -105.5) construction
  arc A212 (6.325, -105.5) -> (9.5, -102.325) centre (6.325, -102.325) ccw
  line L322 (-9.5, -102.325) -> (-9.5, -89.675)
  line L323 (9.5, -89.675) -> (9.5, -102.325)
  line L324 (9.5, -86.5) -> (-9.5, -105.5) construction
  arc A213 (-6.325, -86.5) -> (-9.5, -89.675) centre (-6.325, -89.675) ccw
  arc A214 (9.5, -89.675) -> (6.325, -86.5) centre (6.325, -89.675) ccw
  line L325 (6.325, -105.5) -> (-6.325, -105.5)
  line L326 (-6.325, -86.5) -> (6.325, -86.5)
  arc A215 (-9.5, -102.325) -> (-6.325, -105.5) centre (-6.325, -102.325) ccw
  line L327 (-9.5, -86.5) -> (9.5, -105.5) construction
  arc A216 (30.325, -105.5) -> (33.5, -102.325) centre (30.325, -102.325) ccw
  line L328 (14.5, -102.325) -> (14.5, -89.675)
  line L329 (33.5, -89.675) -> (33.5, -102.325)
  line L330 (33.5, -86.5) -> (14.5, -105.5) construction
  arc A217 (17.675, -86.5) -> (14.5, -89.675) centre (17.675, -89.675) ccw
  arc A218 (33.5, -89.675) -> (30.325, -86.5) centre (30.325, -89.675) ccw
  line L331 (30.325, -105.5) -> (17.675, -105.5)
  line L332 (17.675, -86.5) -> (30.325, -86.5)
  arc A219 (14.5, -102.325) -> (17.675, -105.5) centre (17.675, -102.325) ccw
  line L333 (14.5, -86.5) -> (33.5, -105.5) construction
  arc A220 (54.325, -105.5) -> (57.5, -102.325) centre (54.325, -102.325) ccw
  line L334 (38.5, -102.325) -> (38.5, -89.675)
  line L335 (57.5, -89.675) -> (57.5, -102.325)
  line L336 (57.5, -86.5) -> (38.5, -105.5) construction
  arc A221 (41.675, -86.5) -> (38.5, -89.675) centre (41.675, -89.675) ccw
  arc A222 (57.5, -89.675) -> (54.325, -86.5) centre (54.325, -89.675) ccw
  line L337 (54.325, -105.5) -> (41.675, -105.5)
  line L338 (41.675, -86.5) -> (54.325, -86.5)
  arc A223 (38.5, -102.325) -> (41.675, -105.5) centre (41.675, -102.325) ccw
  line L339 (38.5, -86.5) -> (57.5, -105.5) construction
  arc A224 (78.325, -105.5) -> (81.5, -102.325) centre (78.325, -102.325) ccw
  line L340 (62.5, -102.325) -> (62.5, -89.675)
  line L341 (81.5, -89.675) -> (81.5, -102.325)
  line L342 (81.5, -86.5) -> (62.5, -105.5) construction
  arc A225 (65.675, -86.5) -> (62.5, -89.675) centre (65.675, -89.675) ccw
  arc A226 (81.5, -89.675) -> (78.325, -86.5) centre (78.325, -89.675) ccw
  line L343 (78.325, -105.5) -> (65.675, -105.5)
  line L344 (65.675, -86.5) -> (78.325, -86.5)
  arc A227 (62.5, -102.325) -> (65.675, -105.5) centre (65.675, -102.325) ccw
  line L345 (62.5, -86.5) -> (81.5, -105.5) construction
  arc A228 (102.325, -105.5) -> (105.5, -102.325) centre (102.325, -102.325) ccw
  line L346 (86.5, -102.325) -> (86.5, -89.675)
  line L347 (105.5, -89.675) -> (105.5, -102.325)
  line L348 (105.5, -86.5) -> (86.5, -105.5) construction
  arc A229 (89.675, -86.5) -> (86.5, -89.675) centre (89.675, -89.675) ccw
  arc A230 (105.5, -89.675) -> (102.325, -86.5) centre (102.325, -89.675) ccw
  line L349 (102.325, -105.5) -> (89.675, -105.5)
  line L350 (89.675, -86.5) -> (102.325, -86.5)
  arc A231 (86.5, -102.325) -> (89.675, -105.5) centre (89.675, -102.325) ccw
  line L351 (86.5, -86.5) -> (105.5, -105.5) construction
  arc A232 (126.325, -105.5) -> (129.5, -102.325) centre (126.325, -102.325) ccw
  line L352 (110.5, -102.325) -> (110.5, -89.675)
  line L353 (129.5, -89.675) -> (129.5, -102.325)
  line L354 (129.5, -86.5) -> (110.5, -105.5) construction
  arc A233 (113.675, -86.5) -> (110.5, -89.675) centre (113.675, -89.675) ccw
  arc A234 (129.5, -89.675) -> (126.325, -86.5) centre (126.325, -89.675) ccw
  line L355 (126.325, -105.5) -> (113.675, -105.5)
  line L356 (113.675, -86.5) -> (126.325, -86.5)
  arc A235 (110.5, -102.325) -> (113.675, -105.5) centre (113.675, -102.325) ccw
  line L357 (110.5, -86.5) -> (129.5, -105.5) construction
  arc A236 (150.325, -105.5) -> (153.5, -102.325) centre (150.325, -102.325) ccw
  line L358 (134.5, -102.325) -> (134.5, -89.675)
  line L359 (153.5, -89.675) -> (153.5, -102.325)
  line L360 (153.5, -86.5) -> (134.5, -105.5) construction
  arc A237 (137.675, -86.5) -> (134.5, -89.675) centre (137.675, -89.675) ccw
  arc A238 (153.5, -89.675) -> (150.325, -86.5) centre (150.325, -89.675) ccw
  line L361 (150.325, -105.5) -> (137.675, -105.5)
  line L362 (137.675, -86.5) -> (150.325, -86.5)
  arc A239 (134.5, -102.325) -> (137.675, -105.5) centre (137.675, -102.325) ccw
  line L363 (134.5, -86.5) -> (153.5, -105.5) construction
  arc A240 (174.325, -105.5) -> (177.5, -102.325) centre (174.325, -102.325) ccw
  line L364 (158.5, -102.325) -> (158.5, -89.675)
  line L365 (177.5, -89.675) -> (177.5, -102.325)
  line L366 (177.5, -86.5) -> (158.5, -105.5) construction
  arc A241 (161.675, -86.5) -> (158.5, -89.675) centre (161.675, -89.675) ccw
  arc A242 (177.5, -89.675) -> (174.325, -86.5) centre (174.325, -89.675) ccw
  line L367 (174.325, -105.5) -> (161.675, -105.5)
  line L368 (161.675, -86.5) -> (174.325, -86.5)
  arc A243 (158.5, -102.325) -> (161.675, -105.5) centre (161.675, -102.325) ccw
  line L369 (158.5, -86.5) -> (177.5, -105.5) construction
  arc A244 (-161.675, -81.5) -> (-158.5, -78.325) centre (-161.675, -78.325) ccw
  line L370 (-177.5, -78.325) -> (-177.5, -65.675)
  line L371 (-158.5, -65.675) -> (-158.5, -78.325)
  line L372 (-158.5, -62.5) -> (-177.5, -81.5) construction
  arc A245 (-174.325, -62.5) -> (-177.5, -65.675) centre (-174.325, -65.675) ccw
  arc A246 (-158.5, -65.675) -> (-161.675, -62.5) centre (-161.675, -65.675) ccw
  line L373 (-161.675, -81.5) -> (-174.325, -81.5)
  line L374 (-174.325, -62.5) -> (-161.675, -62.5)
  arc A247 (-177.5, -78.325) -> (-174.325, -81.5) centre (-174.325, -78.325) ccw
  line L375 (-177.5, -62.5) -> (-158.5, -81.5) construction
  arc A248 (-137.675, -81.5) -> (-134.5, -78.325) centre (-137.675, -78.325) ccw
  line L376 (-153.5, -78.325) -> (-153.5, -65.675)
  line L377 (-134.5, -65.675) -> (-134.5, -78.325)
  line L378 (-134.5, -62.5) -> (-153.5, -81.5) construction
  arc A249 (-150.325, -62.5) -> (-153.5, -65.675) centre (-150.325, -65.675) ccw
  arc A250 (-134.5, -65.675) -> (-137.675, -62.5) centre (-137.675, -65.675) ccw
  line L379 (-137.675, -81.5) -> (-150.325, -81.5)
  line L380 (-150.325, -62.5) -> (-137.675, -62.5)
  arc A251 (-153.5, -78.325) -> (-150.325, -81.5) centre (-150.325, -78.325) ccw
  line L381 (-153.5, -62.5) -> (-134.5, -81.5) construction
  arc A252 (-113.675, -81.5) -> (-110.5, -78.325) centre (-113.675, -78.325) ccw
  line L382 (-129.5, -78.325) -> (-129.5, -65.675)
  line L383 (-110.5, -65.675) -> (-110.5, -78.325)
  line L384 (-110.5, -62.5) -> (-129.5, -81.5) construction
  arc A253 (-126.325, -62.5) -> (-129.5, -65.675) centre (-126.325, -65.675) ccw
  arc A254 (-110.5, -65.675) -> (-113.675, -62.5) centre (-113.675, -65.675) ccw
  line L385 (-113.675, -81.5) -> (-126.325, -81.5)
  line L386 (-126.325, -62.5) -> (-113.675, -62.5)
  arc A255 (-129.5, -78.325) -> (-126.325, -81.5) centre (-126.325, -78.325) ccw
  line L387 (-129.5, -62.5) -> (-110.5, -81.5) construction
  arc A256 (-89.675, -81.5) -> (-86.5, -78.325) centre (-89.675, -78.325) ccw
  line L388 (-105.5, -78.325) -> (-105.5, -65.675)
  line L389 (-86.5, -65.675) -> (-86.5, -78.325)
  line L390 (-86.5, -62.5) -> (-105.5, -81.5) construction
  arc A257 (-102.325, -62.5) -> (-105.5, -65.675) centre (-102.325, -65.675) ccw
  arc A258 (-86.5, -65.675) -> (-89.675, -62.5) centre (-89.675, -65.675) ccw
  line L391 (-89.675, -81.5) -> (-102.325, -81.5)
  line L392 (-102.325, -62.5) -> (-89.675, -62.5)
  arc A259 (-105.5, -78.325) -> (-102.325, -81.5) centre (-102.325, -78.325) ccw
  line L393 (-105.5, -62.5) -> (-86.5, -81.5) construction
  arc A260 (-65.675, -81.5) -> (-62.5, -78.325) centre (-65.675, -78.325) ccw
  line L394 (-81.5, -78.325) -> (-81.5, -65.675)
  line L395 (-62.5, -65.675) -> (-62.5, -78.325)
  line L396 (-62.5, -62.5) -> (-81.5, -81.5) construction
  arc A261 (-78.325, -62.5) -> (-81.5, -65.675) centre (-78.325, -65.675) ccw
  arc A262 (-62.5, -65.675) -> (-65.675, -62.5) centre (-65.675, -65.675) ccw
  line L397 (-65.675, -81.5) -> (-78.325, -81.5)
  line L398 (-78.325, -62.5) -> (-65.675, -62.5)
  arc A263 (-81.5, -78.325) -> (-78.325, -81.5) centre (-78.325, -78.325) ccw
  line L399 (-81.5, -62.5) -> (-62.5, -81.5) construction
  arc A264 (-41.675, -81.5) -> (-38.5, -78.325) centre (-41.675, -78.325) ccw
  line L400 (-57.5, -78.325) -> (-57.5, -65.675)
  line L401 (-38.5, -65.675) -> (-38.5, -78.325)
  line L402 (-38.5, -62.5) -> (-57.5, -81.5) construction
  arc A265 (-54.325, -62.5) -> (-57.5, -65.675) centre (-54.325, -65.675) ccw
  arc A266 (-38.5, -65.675) -> (-41.675, -62.5) centre (-41.675, -65.675) ccw
  line L403 (-41.675, -81.5) -> (-54.325, -81.5)
  line L404 (-54.325, -62.5) -> (-41.675, -62.5)
  arc A267 (-57.5, -78.325) -> (-54.325, -81.5) centre (-54.325, -78.325) ccw
  line L405 (-57.5, -62.5) -> (-38.5, -81.5) construction
  arc A268 (-17.675, -81.5) -> (-14.5, -78.325) centre (-17.675, -78.325) ccw
  line L406 (-33.5, -78.325) -> (-33.5, -65.675)
  line L407 (-14.5, -65.675) -> (-14.5, -78.325)
  line L408 (-14.5, -62.5) -> (-33.5, -81.5) construction
  arc A269 (-30.325, -62.5) -> (-33.5, -65.675) centre (-30.325, -65.675) ccw
  arc A270 (-14.5, -65.675) -> (-17.675, -62.5) centre (-17.675, -65.675) ccw
  line L409 (-17.675, -81.5) -> (-30.325, -81.5)
  line L410 (-30.325, -62.5) -> (-17.675, -62.5)
  arc A271 (-33.5, -78.325) -> (-30.325, -81.5) centre (-30.325, -78.325) ccw
  line L411 (-33.5, -62.5) -> (-14.5, -81.5) construction
  arc A272 (6.325, -81.5) -> (9.5, -78.325) centre (6.325, -78.325) ccw
  line L412 (-9.5, -78.325) -> (-9.5, -65.675)
  line L413 (9.5, -65.675) -> (9.5, -78.325)
  line L414 (9.5, -62.5) -> (-9.5, -81.5) construction
  arc A273 (-6.325, -62.5) -> (-9.5, -65.675) centre (-6.325, -65.675) ccw
  arc A274 (9.5, -65.675) -> (6.325, -62.5) centre (6.325, -65.675) ccw
  line L415 (6.325, -81.5) -> (-6.325, -81.5)
  line L416 (-6.325, -62.5) -> (6.325, -62.5)
  arc A275 (-9.5, -78.325) -> (-6.325, -81.5) centre (-6.325, -78.325) ccw
  line L417 (-9.5, -62.5) -> (9.5, -81.5) construction
  arc A276 (30.325, -81.5) -> (33.5, -78.325) centre (30.325, -78.325) ccw
  line L418 (14.5, -78.325) -> (14.5, -65.675)
  line L419 (33.5, -65.675) -> (33.5, -78.325)
  line L420 (33.5, -62.5) -> (14.5, -81.5) construction
  arc A277 (17.675, -62.5) -> (14.5, -65.675) centre (17.675, -65.675) ccw
  arc A278 (33.5, -65.675) -> (30.325, -62.5) centre (30.325, -65.675) ccw
  line L421 (30.325, -81.5) -> (17.675, -81.5)
  line L422 (17.675, -62.5) -> (30.325, -62.5)
  arc A279 (14.5, -78.325) -> (17.675, -81.5) centre (17.675, -78.325) ccw
  line L423 (14.5, -62.5) -> (33.5, -81.5) construction
  arc A280 (54.325, -81.5) -> (57.5, -78.325) centre (54.325, -78.325) ccw
  line L424 (38.5, -78.325) -> (38.5, -65.675)
  line L425 (57.5, -65.675) -> (57.5, -78.325)
  line L426 (57.5, -62.5) -> (38.5, -81.5) construction
  arc A281 (41.675, -62.5) -> (38.5, -65.675) centre (41.675, -65.675) ccw
  arc A282 (57.5, -65.675) -> (54.325, -62.5) centre (54.325, -65.675) ccw
  line L427 (54.325, -81.5) -> (41.675, -81.5)
  line L428 (41.675, -62.5) -> (54.325, -62.5)
  arc A283 (38.5, -78.325) -> (41.675, -81.5) centre (41.675, -78.325) ccw
  line L429 (38.5, -62.5) -> (57.5, -81.5) construction
  arc A284 (78.325, -81.5) -> (81.5, -78.325) centre (78.325, -78.325) ccw
  line L430 (62.5, -78.325) -> (62.5, -65.675)
  line L431 (81.5, -65.675) -> (81.5, -78.325)
  line L432 (81.5, -62.5) -> (62.5, -81.5) construction
  arc A285 (65.675, -62.5) -> (62.5, -65.675) centre (65.675, -65.675) ccw
  arc A286 (81.5, -65.675) -> (78.325, -62.5) centre (78.325, -65.675) ccw
  line L433 (78.325, -81.5) -> (65.675, -81.5)
  line L434 (65.675, -62.5) -> (78.325, -62.5)
  arc A287 (62.5, -78.325) -> (65.675, -81.5) centre (65.675, -78.325) ccw
  line L435 (62.5, -62.5) -> (81.5, -81.5) construction
  arc A288 (102.325, -81.5) -> (105.5, -78.325) centre (102.325, -78.325) ccw
  line L436 (86.5, -78.325) -> (86.5, -65.675)
  line L437 (105.5, -65.675) -> (105.5, -78.325)
  line L438 (105.5, -62.5) -> (86.5, -81.5) construction
  arc A289 (89.675, -62.5) -> (86.5, -65.675) centre (89.675, -65.675) ccw
  arc A290 (105.5, -65.675) -> (102.325, -62.5) centre (102.325, -65.675) ccw
  line L439 (102.325, -81.5) -> (89.675, -81.5)
  line L440 (89.675, -62.5) -> (102.325, -62.5)
  arc A291 (86.5, -78.325) -> (89.675, -81.5) centre (89.675, -78.325) ccw
  line L441 (86.5, -62.5) -> (105.5, -81.5) construction
  arc A292 (126.325, -81.5) -> (129.5, -78.325) centre (126.325, -78.325) ccw
  line L442 (110.5, -78.325) -> (110.5, -65.675)
  line L443 (129.5, -65.675) -> (129.5, -78.325)
  line L444 (129.5, -62.5) -> (110.5, -81.5) construction
  arc A293 (113.675, -62.5) -> (110.5, -65.675) centre (113.675, -65.675) ccw
  arc A294 (129.5, -65.675) -> (126.325, -62.5) centre (126.325, -65.675) ccw
  line L445 (126.325, -81.5) -> (113.675, -81.5)
  line L446 (113.675, -62.5) -> (126.325, -62.5)
  arc A295 (110.5, -78.325) -> (113.675, -81.5) centre (113.675, -78.325) ccw
  line L447 (110.5, -62.5) -> (129.5, -81.5) construction
  arc A296 (150.325, -81.5) -> (153.5, -78.325) centre (150.325, -78.325) ccw
  line L448 (134.5, -78.325) -> (134.5, -65.675)
  line L449 (153.5, -65.675) -> (153.5, -78.325)
  line L450 (153.5, -62.5) -> (134.5, -81.5) construction
  arc A297 (137.675, -62.5) -> (134.5, -65.675) centre (137.675, -65.675) ccw
  arc A298 (153.5, -65.675) -> (150.325, -62.5) centre (150.325, -65.675) ccw
  line L451 (150.325, -81.5) -> (137.675, -81.5)
  line L452 (137.675, -62.5) -> (150.325, -62.5)
  arc A299 (134.5, -78.325) -> (137.675, -81.5) centre (137.675, -78.325) ccw
  line L453 (134.5, -62.5) -> (153.5, -81.5) construction
  arc A300 (174.325, -81.5) -> (177.5, -78.325) centre (174.325, -78.325) ccw
  line L454 (158.5, -78.325) -> (158.5, -65.675)
  line L455 (177.5, -65.675) -> (177.5, -78.325)
  line L456 (177.5, -62.5) -> (158.5, -81.5) construction
  arc A301 (161.675, -62.5) -> (158.5, -65.675) centre (161.675, -65.675) ccw
  arc A302 (177.5, -65.675) -> (174.325, -62.5) centre (174.325, -65.675) ccw
  line L457 (174.325, -81.5) -> (161.675, -81.5)
  line L458 (161.675, -62.5) -> (174.325, -62.5)
  arc A303 (158.5, -78.325) -> (161.675, -81.5) centre (161.675, -78.325) ccw
  line L459 (158.5, -62.5) -> (177.5, -81.5) construction
  arc A304 (-161.675, -57.5) -> (-158.5, -54.325) centre (-161.675, -54.325) ccw
  line L460 (-177.5, -54.325) -> (-177.5, -41.675)
  line L461 (-158.5, -41.675) -> (-158.5, -54.325)
  line L462 (-158.5, -38.5) -> (-177.5, -57.5) construction
  arc A305 (-174.325, -38.5) -> (-177.5, -41.675) centre (-174.325, -41.675) ccw
  arc A306 (-158.5, -41.675) -> (-161.675, -38.5) centre (-161.675, -41.675) ccw
  line L463 (-161.675, -57.5) -> (-174.325, -57.5)
  line L464 (-174.325, -38.5) -> (-161.675, -38.5)
  arc A307 (-177.5, -54.325) -> (-174.325, -57.5) centre (-174.325, -54.325) ccw